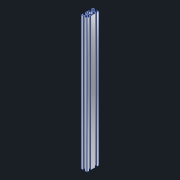
# Autodesk Inventor part: KNFS5-2040_2
Saved by Autodesk Inventor 2022 (Build 260153000, 153)
## iProperties
Category: PARTsolutions
Company: MISUMI
Part Number: KNFS5-2040_2
Material: アルミニウム 6061
Catalog Web Link: www.cadenas.de
Description: KHFS5-2040, KHFSB5-2040, KCAF5-2040, KNFS5-2040, KHFSY5-2040-Aluminum Frames -5 Series-2Row Groove 20x40 mm Square -Fixed Length
Vendor: MISUMI
Document SubType Name: Modeling
Designer: partserver
Manufacturer: MISUMI
Mass: 278.585 g
Surface Area: 1013.22 cm^2
Volume: 103.18 cm^3
Density: 2.7 g/cm^3
Appearance: アルミニウム - フラット
L: 4000
PSOL_IDENT_0: {$CADENAS_DATA\23d-libs\misumi\metric\38_al_extrusions_blackets\5\khfs5_2040.prj},225 {VTYP=3D},{NB=
PSOL_IDENT_1: KNFS5-2040-4000},{LINA=KNFS5-2040-4000},{NN=KHFS5-2040, KHFSB5-2040, KCAF5-2040, KNFS5-2040, KHFSY5-
PSOL_IDENT_2: 2040},{DATE=19.08.2021 01:58:42},{GEOMDATE=11.08.2021 05:35:50},{VERSION=},{LINEID=570},{WBVAR=},{WB
PSOL_IDENT_3: NUMERIC=}  {NB=KNFS5-2040-4000},{LINA=KNFS5-2040-4000},{KT=9},{PN=KNFS5-2040-4000},{TPS=KNFS5-2040},
PSOL_IDENT_4: {TP=KNFS5},{FRM=2040},{FEAT=Four-Side Slots},{L=4000},{LTOL=+/- 0.5},{MASS=0},{SA=153},{GMILX=0.57x1
PSOL_IDENT_5: 0^4},{GMILY=0.57x10^4},{CLF=NFS5-2040},{WIDTH=40.000},{HEIGHT=20.000},{VER=2},{DIM=9},{DRILLDIA=4.20
PSOL_IDENT_6: 0},{FRMW=20.000},{FRMH=40.000},{FRD=4.200},{COLOR=}
NB: KNFS5-2040-4000
NN: KHFS5-2040, KHFSB5-2040, KCAF5-2040, KNFS5-2040, KHFSY5-2040
NT: Aluminum Frames -5 Series-2Row Groove 20x40 mm Square -Fixed Length
NBSYN: $PN.
LINA: KNFS5-2040-4000
CATALOG: Misumi
PN: KNFS5-2040-4000
TPS: KNFS5-2040
SUPPLIER: MISUMI
ARTICLENO: KNFS5-2040-4000
BOMINFO: KNFS5-2040-4000
CREATOR: CADENAS GmbH
Title: KNFS5-2040-4000
Author: Cadenas PARTsolutions
Comments: Aluminum Frames -5 Series-2Row Groove 20x40 mm Square -Fixed Length
Autodesk Inventor part; units mm, degrees
ref_plane "YZ Plane" through (0, 0, 0) normal (1, 0, 0) x (0, 1, 0)
ref_plane "XZ Plane" through (0, 0, 0) normal (0, 1, 0) x (-1, 0, 0)
ref_plane "XY Plane" through (0, 0, 0) normal (0, 0, 1) x (1, 0, 0)
sketch "_____4" plane through (0, 0, 0) normal (0, 0, 1) x (1, 0, 0)
  line L0 (-10, -7) -> (-8, -7)
  line L1 (-8, -7) -> (-8, -4)
  line L2 (-8, -4) -> (-7.0607, -4)
  line L3 (-7.0607, -4) -> (-4, -7.0607)
  line L4 (-4, -7.0607) -> (-4, -7.5)
  line L5 (-4, -7.5) -> (-3.751, -8.7811)
  line L6 (-3.751, -8.7811) -> (-3.933, -9.0964)
  arc A0 (-3.933, -9.0964) -> (-3.933, -9.5964) centre (-3.5, -9.3464) ccw
  line L7 (-3.933, -9.5964) -> (-3.7, -10)
  line L8 (-3.7, -10) -> (-3.933, -10.4036)
  arc A1 (-3.933, -10.4036) -> (-4, -10.6536) centre (-3.5, -10.6536) ccw
  line L9 (-4, -10.6536) -> (-4, -12.9393)
  line L10 (-4, -12.9393) -> (-7.0607, -16)
  line L11 (-7.0607, -16) -> (-8, -16)
  line L12 (-8, -16) -> (-8, -13)
  line L13 (-8, -13) -> (-10, -13)
  line L14 (-10, -13) -> (-10, -19)
  arc A2 (-10, -19) -> (-9, -20) centre (-9, -19) ccw
  line L15 (-9, -20) -> (-3, -20)
  line L16 (-3, -20) -> (-3, -18)
  line L17 (-3, -18) -> (-6, -18)
  line L18 (-6, -18) -> (-6, -17.0607)
  line L19 (-6, -17.0607) -> (-2.9393, -14)
  line L20 (-2.9393, -14) -> (-2.5, -14)
  line L21 (-2.5, -14) -> (-1.2189, -13.751)
  line L22 (-1.2189, -13.751) -> (-0.9036, -13.933)
  arc A3 (-0.9036, -13.933) -> (-0.4036, -13.933) centre (-0.6536, -13.5) ccw
  line L23 (-0.4036, -13.933) -> (0, -13.7)
  line L24 (0, -13.7) -> (0.4036, -13.933)
  arc A4 (0.4036, -13.933) -> (0.6536, -14) centre (0.6536, -13.5) ccw
  line L25 (0.6536, -14) -> (2.9393, -14)
  line L26 (2.9393, -14) -> (6, -17.0607)
  line L27 (6, -17.0607) -> (6, -18)
  line L28 (6, -18) -> (3, -18)
  line L29 (3, -18) -> (3, -20)
  line L30 (3, -20) -> (9, -20)
  arc A5 (9, -20) -> (10, -19) centre (9, -19) ccw
  line L31 (10, -19) -> (10, -13)
  line L32 (10, -13) -> (8, -13)
  line L33 (8, -13) -> (8, -16)
  line L34 (8, -16) -> (7.0607, -16)
  line L35 (7.0607, -16) -> (4, -12.9393)
  line L36 (4, -12.9393) -> (4, -12.5)
  line L37 (4, -12.5) -> (3.751, -11.2189)
  line L38 (3.751, -11.2189) -> (3.933, -10.9036)
  arc A6 (3.933, -10.9036) -> (3.933, -10.4036) centre (3.5, -10.6536) ccw
  line L39 (3.933, -10.4036) -> (3.7, -10)
  line L40 (3.7, -10) -> (3.933, -9.5964)
  arc A7 (3.933, -9.5964) -> (4, -9.3464) centre (3.5, -9.3464) ccw
  line L41 (4, -9.3464) -> (4, -7.0607)
  line L42 (4, -7.0607) -> (7.0607, -4)
  line L43 (7.0607, -4) -> (8, -4)
  line L44 (8, -4) -> (8, -7)
  line L45 (8, -7) -> (10, -7)
  line L46 (10, -7) -> (10, 7)
  line L47 (10, 7) -> (8, 7)
  line L48 (8, 7) -> (8, 4)
  line L49 (8, 4) -> (7.0607, 4)
  line L50 (7.0607, 4) -> (4, 7.0607)
  line L51 (4, 7.0607) -> (4, 9.3464)
  arc A8 (4, 9.3464) -> (3.933, 9.5964) centre (3.5, 9.3464) ccw
  line L52 (3.933, 9.5964) -> (3.7, 10)
  line L53 (3.7, 10) -> (3.933, 10.4036)
  arc A9 (3.933, 10.4036) -> (3.933, 10.9036) centre (3.5, 10.6536) ccw
  line L54 (3.933, 10.9036) -> (3.751, 11.2189)
  line L55 (3.751, 11.2189) -> (4, 12.5)
  line L56 (4, 12.5) -> (4, 12.9393)
  line L57 (4, 12.9393) -> (7.0607, 16)
  line L58 (7.0607, 16) -> (8, 16)
  line L59 (8, 16) -> (8, 13)
  line L60 (8, 13) -> (10, 13)
  line L61 (10, 13) -> (10, 19)
  arc A10 (10, 19) -> (9, 20) centre (9, 19) ccw
  line L62 (9, 20) -> (3, 20)
  line L63 (3, 20) -> (3, 18)
  line L64 (3, 18) -> (6, 18)
  line L65 (6, 18) -> (6, 17.0607)
  line L66 (6, 17.0607) -> (2.9393, 14)
  line L67 (2.9393, 14) -> (0.6536, 14)
  arc A11 (0.6536, 14) -> (0.4036, 13.933) centre (0.6536, 13.5) ccw
  line L68 (0.4036, 13.933) -> (0, 13.7)
  line L69 (0, 13.7) -> (-0.4036, 13.933)
  arc A12 (-0.4036, 13.933) -> (-0.9036, 13.933) centre (-0.6536, 13.5) ccw
  line L70 (-0.9036, 13.933) -> (-1.2189, 13.751)
  line L71 (-1.2189, 13.751) -> (-2.5, 14)
  line L72 (-2.5, 14) -> (-2.9393, 14)
  line L73 (-2.9393, 14) -> (-6, 17.0607)
  line L74 (-6, 17.0607) -> (-6, 18)
  line L75 (-6, 18) -> (-3, 18)
  line L76 (-3, 18) -> (-3, 20)
  line L77 (-3, 20) -> (-9, 20)
  arc A13 (-9, 20) -> (-10, 19) centre (-9, 19) ccw
  line L78 (-10, 19) -> (-10, 13)
  line L79 (-10, 13) -> (-8, 13)
  line L80 (-8, 13) -> (-8, 16)
  line L81 (-8, 16) -> (-7.0607, 16)
  line L82 (-7.0607, 16) -> (-4, 12.9393)
  line L83 (-4, 12.9393) -> (-4, 10.6536)
  arc A14 (-4, 10.6536) -> (-3.933, 10.4036) centre (-3.5, 10.6536) ccw
  line L84 (-3.933, 10.4036) -> (-3.7, 10)
  line L85 (-3.7, 10) -> (-3.933, 9.5964)
  arc A15 (-3.933, 9.5964) -> (-3.933, 9.0964) centre (-3.5, 9.3464) ccw
  line L86 (-3.933, 9.0964) -> (-3.751, 8.7811)
  line L87 (-3.751, 8.7811) -> (-4, 7.5)
  line L88 (-4, 7.5) -> (-4, 7.0607)
  line L89 (-4, 7.0607) -> (-7.0607, 4)
  line L90 (-7.0607, 4) -> (-8, 4)
  line L91 (-8, 4) -> (-8, 7)
  line L92 (-8, 7) -> (-10, 7)
  line L93 (-10, 7) -> (-10, -7)
  line L94 (-8, 1.7) -> (-8, -1.7)
  arc A16 (-8, -1.7) -> (-7.7, -2) centre (-7.7, -1.7) ccw
  line L95 (-7.7, -2) -> (-7.0636, -2)
  arc A17 (-6.8515, -2.0879) -> (-7.0636, -2) centre (-7.0636, -2.3) ccw
  line L96 (-6.8515, -2.0879) -> (-2.9393, -6)
  line L97 (-2.9393, -6) -> (2.9393, -6)
  line L98 (2.9393, -6) -> (6.8515, -2.0879)
  arc A18 (7.0636, -2) -> (6.8515, -2.0879) centre (7.0636, -2.3) ccw
  line L99 (7.0636, -2) -> (7.7, -2)
  arc A19 (7.7, -2) -> (8, -1.7) centre (7.7, -1.7) ccw
  line L100 (8, -1.7) -> (8, 1.7)
  arc A20 (8, 1.7) -> (7.7, 2) centre (7.7, 1.7) ccw
  line L101 (7.7, 2) -> (7.0636, 2)
  arc A21 (6.8515, 2.0879) -> (7.0636, 2) centre (7.0636, 2.3) ccw
  line L102 (6.8515, 2.0879) -> (2.9393, 6)
  line L103 (2.9393, 6) -> (-2.9393, 6)
  line L104 (-2.9393, 6) -> (-6.8515, 2.0879)
  arc A22 (-7.0636, 2) -> (-6.8515, 2.0879) centre (-7.0636, 2.3) ccw
  line L105 (-7.0636, 2) -> (-7.7, 2)
  arc A23 (-7.7, 2) -> (-8, 1.7) centre (-7.7, 1.7) ccw
  constraints: 212 end point, 48 point on circle, 24 centre point
extrude "Extrusion1" add sketch "_____4" against normal blind 445
sketch "Sketch2" plane through (0, 0, -445) normal (0, 0, -1) x (-1, 0, 0)
  point P0 (0, 10)
hole "Hole1" at (0, 10, -445) direction (0, 0, 1) diameter 4.2 depth 4000
sketch "Sketch3" plane through (0, 0, 0) normal (0, 0, 1) x (1, 0, 0)
  point P0 (0, -10)
hole "Hole2" at (0, -10, 0) direction (0, 0, -1) diameter 4.2 depth 4000
body "Solid1"
